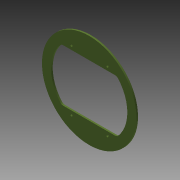
# Autodesk Inventor part: Light Sensor PCB
Saved by Autodesk Inventor 2015 (Build 190159000, 159)
## iProperties
Created: 2016-10-14
Part Number: Light Sensor PCB
Material: Generic
Document SubType Name: Modeling
Designer: James Yelland
Density: 1 g/cm^3
Appearance: Default
Author: James Yelland
Autodesk Inventor part; units mm, degrees
ref_plane "YZ Plane" through (0, 0, 0) normal (1, 0, 0) x (0, 1, 0)
ref_plane "XZ Plane" through (0, 0, 0) normal (0, 1, 0) x (-1, 0, 0)
ref_plane "XY Plane" through (0, 0, 0) normal (0, 0, 1) x (1, 0, 0)
sketch "Sketch1" plane through (0, 0, 0) normal (0, 1, 0) x (-1, 0, 0)
  circle A0 centre (0, 0) radius 59.5
  line L0 (0, 33) -> (-32.6343, 33)
  line L1 (0, 33) -> (32.6343, 33)
  line L2 (0, -33) -> (-32.6343, -33)
  line L3 (0, -33) -> (32.6343, -33)
  arc A1 (-36.429, 31.2558) -> (-36.429, -31.2558) centre (0, 0) ccw
  arc A2 (36.429, -31.2558) -> (36.429, 31.2558) centre (0, 0) ccw
  arc A3 (36.429, 31.2558) -> (32.6343, 33) centre (32.6343, 28) ccw
  arc A4 (-32.6343, 33) -> (-36.429, 31.2558) centre (-32.6343, 28) ccw
  arc A5 (-36.429, -31.2558) -> (-32.6343, -33) centre (-32.6343, -28) ccw
  arc A6 (32.6343, -33) -> (36.429, -31.2558) centre (32.6343, -28) ccw
  line L4 (32.6343, 33) -> (22.6343, 33)
  circle A7 centre (22.6343, 38) radius 1.6
  line L5 (0, 0) -> (0, 10.7969)
  line L6 (0, 0) -> (10.7386, 0)
  circle A8 centre (-22.6343, 38) radius 1.6
  circle A9 centre (22.6343, -38) radius 1.6
  circle A10 centre (-22.6343, -38) radius 1.6
  point P0 (-34.8569, 33)
  point P1 (34.8569, 33)
  point P2 (-34.8569, -33)
  point P3 (34.8569, -33)
  dimension "d1" = 119
  dimension "d7" = 5
  dimension "d8" = 10
  dimension "d11" = 3.2
  constraints: 16 point on circle, 14 end point, 11 centre point, 8 tangent, 6 point on line, 3 equal radius, 3 symmetric about line, 2 coincident, 2 horizontal, 1 vertical, 3 other
  measures "d1" diameter of A0
  measures "d7" radius of A3
  measures "d8" distance of L1.end L4.end
  measures "d11" diameter of A7
extrude "Extrusion1" add sketch "Sketch1" along normal blind 2
body "Solid1"
